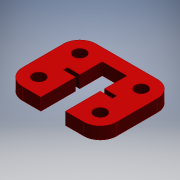
# Autodesk Inventor part: LegMount
Saved by Autodesk Inventor 2016 (Build 200138000, 138)
## iProperties
Created: 2015-12-10
Part Number: LegMount
Material: Generic
Document SubType Name: Modeling
Designer: lk8187
Density: 1 g/cm^3
Appearance: Smooth - Burnt Red
Author: lk8187
Autodesk Inventor part; units mm, degrees
ref_plane "YZ Plane" through (0, 0, 0) normal (1, 0, 0) x (0, 1, 0)
ref_plane "XZ Plane" through (0, 0, 0) normal (0, 1, 0) x (-1, 0, 0)
ref_plane "XY Plane" through (0, 0, 0) normal (0, 0, 1) x (1, 0, 0)
sketch "Sketch1" plane through (0, 0, 0) normal (0, 0, 1) x (1, 0, 0)
  line L0 (-3, -9) -> (-3, -0.5)
  line L1 (-3, -0.5) -> (-6, -0.5)
  line L2 (-6, -0.5) -> (-6, 0.5)
  line L3 (-6, 0.5) -> (-3, 0.5)
  line L4 (-3, 0.5) -> (-3, 6)
  line L5 (-3, 6) -> (3, 6)
  line L6 (3, 6) -> (3, 0.5)
  line L7 (3, 0.5) -> (6, 0.5)
  line L8 (6, 0.5) -> (6, -0.5)
  line L9 (6, -0.5) -> (3, -0.5)
  line L10 (3, -0.5) -> (3, -9)
  line L11 (3, -9) -> (7.5, -9)
  arc A0 (7.5, -9) -> (11.5, -5) centre (7.5, -5) ccw
  line L12 (11.5, -5) -> (11.5, 5)
  arc A1 (11.5, 5) -> (7.5, 9) centre (7.5, 5) ccw
  line L13 (7.5, 9) -> (-7.5, 9)
  arc A2 (-7.5, 9) -> (-11.5, 5) centre (-7.5, 5) ccw
  line L14 (-11.5, 5) -> (-11.5, -5)
  arc A3 (-11.5, -5) -> (-7.5, -9) centre (-7.5, -5) ccw
  line L15 (-7.5, -9) -> (-3, -9)
  circle A4 centre (-7.5, 5) radius 1.5
  circle A5 centre (-7.5, -5) radius 1.5
  circle A6 centre (7.5, -5) radius 1.5
  circle A7 centre (7.5, 5) radius 1.5
  point P0 (0, 0)
  constraints: 32 end point, 8 centre point, 8 point on circle
extrude "Extrusion1" add sketch "Sketch1" along normal blind 3
body "Solid1"
